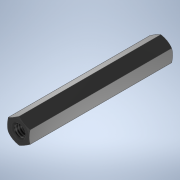
# Autodesk Inventor part: ABLSBF6-39.5-M4-N4
Saved by Autodesk Inventor 2022 (Build 260153000, 153)
## iProperties
Part Number: ABLSBF6-39.5-M4-N4
Material: アルミニウム 2014-T4
Document SubType Name: Modeling
Designer: Masato Kubotera
Density: 2.8 g/cm^3
Appearance: 光沢 - 黒
Catalog Web Link: https://jp.misumi-ec.com/vona2/detail/110300206620/?HissuCode=ABLSBF6-39.5-M4-N4
Description: ReadyMade
Mass: 7.65 g
Surface Area: 11.1939 cm^2
Volume: 1.02926 cm^3
Author: Masato Kubotera
Comments: Width across flats : 6
Autodesk Inventor part; units mm, degrees
ref_plane "YZ Plane" through (0, 0, 0) normal (1, 0, 0) x (0, 1, 0)
ref_plane "XZ Plane" through (0, 0, 0) normal (0, 1, 0) x (-1, 0, 0)
ref_plane "XY Plane" through (0, 0, 0) normal (0, 0, 1) x (1, 0, 0)
sketch "スケッチ1" plane through (0, 0, 0) normal (1, 0, 0) x (0, 1, 0)
  line L0 (-19.75, 0) -> (19.75, 0)
  line L1 (0, 0) -> (0, 3.4641) construction
  line L2 (-19.4821, 3.4641) -> (-19.75, 3)
  line L3 (-19.75, 3) -> (-19.75, 0)
  line L4 (-19.4821, 3.4641) -> (19.4821, 3.4641)
  line L5 (19.4821, 3.4641) -> (19.75, 3)
  line L6 (19.75, 3) -> (19.75, 0)
  dimension "d1" = 3
  dimension "d2" = 3.4641
  dimension "d3" = 30
  dimension "d4" = 39.5
  constraints: 14 end point, 3 perpendicular, 2 midpoint, 1 coincident, 1 horizontal, 1 symmetric about line
  measures "d1" distance of L0.start L2.end
  measures "d2" vertical distance of L0.start L2.start
  measures "d3" angle of L3 L2
  measures "d4" distance of L0.start L0.end
revolve "回転1" add sketch "スケッチ1" angle 360 about axis through (0, -19.75, 0) along (0, 1, 0)
sketch "スケッチ2" plane through (0, 19.75, 0) normal (0, 1, 0) x (1, 0, 0)
  circle A0 centre (0, 0) radius 3.4641 projected
  line L0 (0, -3.4641) -> (-3, -1.7321)
  line L1 (-3, -1.7321) -> (-3, 1.7321)
  line L2 (-3, 1.7321) -> (0, 3.4641)
  line L3 (0, 3.4641) -> (3, 1.7321)
  line L4 (3, 1.7321) -> (3, -1.7321)
  line L5 (3, -1.7321) -> (0, -3.4641)
  point P0 (0, 0)
  point P1 (0, 0)
  point P2 (3, -1.7321)
  point P3 (3, -1.7321)
  point P4 (3, 1.7321)
  point P5 (3, 1.7321)
  point P6 (0, 3.4641)
  point P7 (0, 3.4641)
  point P8 (-3, 1.7321)
  point P9 (-3, 1.7321)
  point P10 (-3, -1.7321)
  point P11 (-3, -1.7321)
  point P12 (0, 0)
  constraints: 12 end point, 2 coincident, 1 vertical, 15 other
extrude "押し出し1" cut sketch "スケッチ2" against normal through all contours A0 L4 | L3 A0 | A0 L5 | L2 A0 | A0 L0 | L1 A0
hole "穴1" at (0, 19.75, 0) direction (0, -1, 0) diameter 3.242 depth 11.8 tip angle 118 countersink diameter 4 countersink angle 90 thread size "M4x0.7" class "6H" standard "ISO Metric profile"
mirror "ミラー1" about plane through (0, 0, 0) normal (0, 1, 0) of "穴1"
equation "\"d2\" = 1.1547 * d1"
